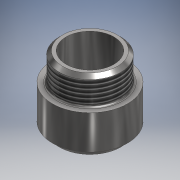
# Autodesk Inventor part: 液压杆盖
Saved by Autodesk Inventor 2019 (Build 230136000, 136)
## iProperties
Created: 2018-12-13
Part Number: 液压杆盖
Material: 不锈钢
Document SubType Name: Modeling
Designer: Administrator
Density: 8 g/cm^3
Appearance: 半抛光
Author: Administrator
Autodesk Inventor part; units mm, degrees
ref_plane "YZ Plane" through (0, 0, 0) normal (1, 0, 0) x (0, 1, 0)
ref_plane "XZ Plane" through (0, 0, 0) normal (0, 1, 0) x (-1, 0, 0)
ref_plane "XY Plane" through (0, 0, 0) normal (0, 0, 1) x (1, 0, 0)
sketch "草图1" plane through (0, 0, 0) normal (0, 1, 0) x (-1, 0, 0)
  circle A0 centre (0, 0) radius 55
  dimension "d0" = 110
  constraints: 1 centre point, 1 coincident
  measures "d0" diameter of A0
extrude "拉伸1" add sketch "草图1" along normal blind 100
sketch "草图2" plane through (0, 100, 0) normal (0, 1, 0) x (1, 0, 0)
  circle A0 centre (0, 0) radius 35
  dimension "d3" = 70
  constraints: 1 centre point, 1 coincident
  measures "d3" diameter of A0
extrude "拉伸2" cut sketch "草图2" against normal blind 100
sketch "草图3" plane through (0, 100, 0) normal (0, 1, 0) x (1, 0, 0)
  circle A0 centre (0, 0) radius 45
  circle A1 centre (0, 0) radius 55
  dimension "d6" = 90
  dimension "d7" = 110
  constraints: 2 centre point, 2 coincident
  measures "d6" diameter of A0
  measures "d7" diameter of A1
extrude "拉伸3" cut sketch "草图3" against normal blind 40
thread "螺纹1" size "M90x6" class "6g" standard "ANSI Metric M Profile" full length
chamfer "倒角1" distance 10 angle 45 1 edges at (55, 0, 0)
chamfer "倒角2" distance 5 angle 45 1 edges at (-45, 100, 0)
fillet "圆角1" radius 3 1 edges at (-45, 60, 0)
